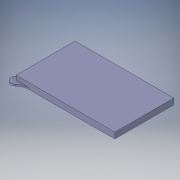
# Autodesk Inventor part: stamp5x3
Saved by Autodesk Inventor 2019 (Build 230136000, 136)
## iProperties
Created: 2019-02-19
Part Number: stamp5x3
Material: PET Plastic
Document SubType Name: Modeling
Designer: jmc
Density: 1.541 g/cm^3
Appearance: Slate Blue
Author: jmc
Autodesk Inventor part; units mm, degrees
ref_plane "YZ Plane" through (0, 0, 0) normal (1, 0, 0) x (0, 1, 0)
ref_plane "XZ Plane" through (0, 0, 0) normal (0, 1, 0) x (-1, 0, 0)
ref_plane "XY Plane" through (0, 0, 0) normal (0, 0, 1) x (1, 0, 0)
sketch "Sketch1" plane through (0, 0, 0) normal (0, 1, 0) x (-1, 0, 0)
  line L0 (24.925, 14.925) -> (-24.925, 14.925)
  line L1 (-24.925, 14.925) -> (-24.925, -14.925)
  line L2 (-24.925, -14.925) -> (24.925, -14.925)
  line L3 (24.925, 14.925) -> (-24.925, -14.925) construction
  line L4 (-24.925, 14.925) -> (24.925, -14.925) construction
  line L5 (24.925, -14.925) -> (24.925, 14.925)
  line L6 (24.925, 5) -> (24.925, 14.925)
  point P0 (0, 0)
  dimension "d0" = 49.85
  dimension "d1" = 29.85
  constraints: 14 end point, 3 parallel, 2 midpoint, 1 horizontal, 1 perpendicular
  measures "d0" distance of L2.end L1.end
  measures "d1" distance of L1.end L0.end
extrude "Extrusion1" add sketch "Sketch1" along normal blind 3
sketch "Sketch2" plane through (0, 0, 0) normal (0, -1, 0) x (1, 0, 0)
  line L0 (-24.925, -14.925) -> (-24.925, 14.925) projected
  arc A0 (-23.2879, 16.8144) -> (-26.5141, 12.995) centre (-24.925, 14.925) ccw
  arc A1 (-24.925, 9.6282) -> (-26.5141, 12.995) centre (-29.2863, 9.6282) ccw
  line L1 (-24.925, 14.925) -> (24.925, 14.925) projected
  arc A2 (-23.2879, 16.8144) -> (-18.2222, 14.925) centre (-18.2222, 22.6605) ccw
  line L2 (-24.925, 14.925) -> (-24.925, -14.925) projected
  point P0 (0, 0)
  dimension "d5" = 5
  constraints: 6 point on circle, 4 tangent, 3 centre point, 2 point on line
  measures "d5" diameter of A0
extrude "Extrusion2" add sketch "Sketch2" against normal blind 0.8
body "Solid1"
